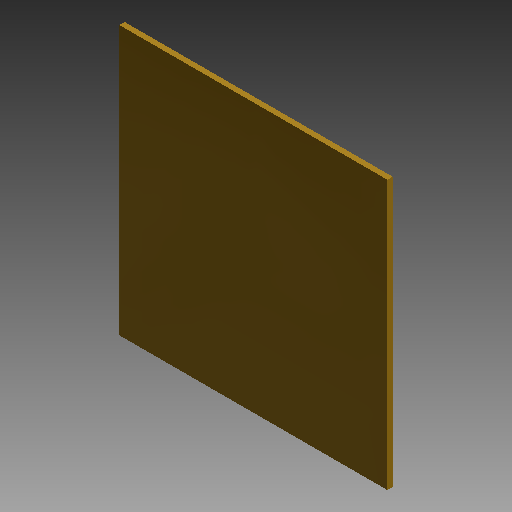
# Autodesk Inventor part: FIDUCIAL
Saved by Autodesk Inventor 2018.2 (Build 222227000, 227)
## iProperties
Part Number: FIDUCIAL
Material: Generic
Document SubType Name: Modeling
Designer: autocad
Appearance: FIDUCIAL-1X2, FIDUCIAL
Author: autocad
Autodesk Inventor part; units mm, degrees
ref_plane "YZ Plane" through (0, 0, 0) normal (1, 0, 0) x (0, 1, 0)
ref_plane "XZ Plane" through (0, 0, 0) normal (0, 1, 0) x (-1, 0, 0)
ref_plane "XY Plane" through (0, 0, 0) normal (0, 0, 1) x (1, 0, 0)
sketch "FIDUCIAL-1X2, FIDUCIAL_155" plane through (0, 0, 0) normal (0, 0, 1) x (1, 0, 0)
  line L0 (0.5082, -0.5069) -> (-0.5039, -0.5069)
  line L1 (-0.5039, -0.5069) -> (-0.5039, 0.5072)
  line L2 (-0.5039, 0.5072) -> (0.5082, 0.5072)
  line L3 (0.5082, 0.5072) -> (0.5082, -0.5069)
  constraints: 8 end point
extrude "Extrusion1" add sketch "FIDUCIAL-1X2, FIDUCIAL_155" along normal blind 0.02
body "Solid1"
